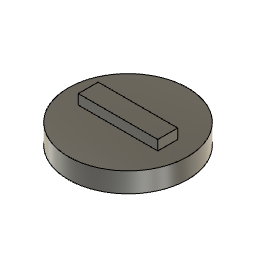
menuButtons v4 (Autodesk Fusion 360 design; units mm, degrees)
Autodesk Fusion 360 part; units mm, degrees
sketch "Sketch1" plane through (0, 0, 0) normal (0, 0, 1) x (1, 0, 0)
  circle A0 centre (0, 0) radius 6
  dimension "d1" = 12
  constraint coincident A0.centre origin
  measures "d1" diameter of A0
extrude "Extrude1" add sketch "Sketch1" along normal blind 2 makes body 1
sketch "Sketch2" plane through (0, 0, 2) normal (0, 0, 1) x (-1, 0, 0)
  circle A0 centre (0, 0) radius 6
  line L0 (-4, 1) -> (4, 1)
  line L1 (4, 1) -> (4, -1)
  line L2 (4, -1) -> (-4, -1)
  line L3 (-4, -1) -> (-4, 1)
  constraint horizontal L0
  constraint vertical L1
  constraint horizontal L2
  constraint vertical L3
extrude "Extrude3" add sketch "Sketch2" along normal blind 1 separate body contours L0 L1 L2 L3 makes body 2
sketch "Sketch3" plane through (0, 0, 2) normal (0, 0, 1) x (-1, 0, 0)
  circle A0 centre (0, 0) radius 6
  line L0 (-1, 1) -> (1, 1)
  line L1 (1, 1) -> (1, -4)
  line L2 (1, -4) -> (-1, -4)
  line L3 (-1, -4) -> (-1, 1)
  line L4 (1, -1) -> (-4, -1)
  line L5 (-4, -1) -> (-4, 1)
  line L6 (-4, 1) -> (1, 1)
  line L7 (1, 1) -> (1, -1)
  line L8 (-1, -1) -> (1, -1)
  line L9 (1, -1) -> (1, 4)
  line L10 (1, 4) -> (-1, 4)
  line L11 (-1, 4) -> (-1, -1)
  line L12 (-1, -1) -> (4, -1)
  line L13 (4, -1) -> (4, 1)
  line L14 (4, 1) -> (-1, 1)
  line L15 (-1, 1) -> (-1, -1)
  constraint horizontal L0
  constraint vertical L1
  constraint horizontal L2
  constraint vertical L3
  constraint horizontal L4
  constraint vertical L5
  constraint horizontal L6
  constraint vertical L7
  constraint coincident L1 L4.start
  constraint horizontal L8
  constraint vertical L9
  constraint horizontal L10
  constraint vertical L11
  constraint coincident L4 L8.start
  constraint coincident L3 L8.start
  constraint horizontal L12
  constraint vertical L13
  constraint horizontal L14
  constraint vertical L15
extrude "Extrude4" add sketch "Sketch3" along normal blind 1 separate body contours L0 L6 L9 L10 L11 L14 | L0 L1 L3 L4 L6 L7 L8 L9 L11 L12 L14 L15 | L3 L4 L5 L6 L11 L15 | L1 L7 L9 L12 L13 L14 | L1 L2 L3 L4 L8 L12 makes body 3
sketch "Sketch4" plane through (0, 0, 2) normal (0, 0, 1) x (-1, 0, 0)
  circle A0 centre (0, 0) radius 6
  line L0 (4, 1) -> (-1, 1)
  line L1 (-1, -1) -> (4, -1)
  line L2 (4, -1) -> (4, 1)
  line L3 (-4, 0) -> (-1.5, -2.5)
  line L4 (-1.5, -2.5) -> (0.5, -2.5)
  line L5 (-4, 0) -> (-1.5, 2.5)
  line L6 (-1.5, 2.5) -> (0.5, 2.5)
  line L7 (0.5, -2.5) -> (-1, -1)
  line L8 (0.5, 2.5) -> (-1, 1)
  constraint horizontal L0
  constraint horizontal L1
  constraint vertical L2
  constraint horizontal L4
  constraint perpendicular L3 L5
  constraint horizontal L6
extrude "Extrude5" add sketch "Sketch4" along normal blind 1 separate body contours L0 L1 L2 L3 L4 L5 L6 L7 L8 makes body 4
copy_body "CopyPasteBodies1" bodies 4 makes body 5
move_body "Move1" bodies 5 to x (-1, 0, 0) y (0, 1, 0) z (0, 0, -1) at (0, 0, 5)
copy_body "CopyPasteBodies2" bodies 1 makes body 6
copy_body "CopyPasteBodies3" bodies 1 makes body 7
copy_body "CopyPasteBodies4" bodies 1 makes body 8
combine "Combine1" operation add target body 2 tool bodies 1
combine "Combine2" operation add target body 3 tool bodies 6
combine "Combine3" operation add target body 4 tool bodies 7
combine "Combine4" operation add target body 5 tool bodies 8
extrude "Extrude2" [suppressed]
hidden bodies 3 4 5
named bodies: "button", "Minus", "Plus", "Right", "Left", "button (1)", "button (1) (1)", "button (2)"
